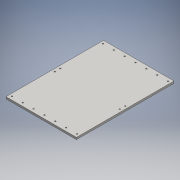
# Autodesk Inventor part: KrackenPlate1
Saved by Autodesk Inventor 2016 (Build 200138000, 138)
## iProperties
Created: 2015-09-06
Part Number: KrackenPlate1
Material: Generic
Document SubType Name: Modeling
Designer: Tim
Density: 1 g/cm^3
Appearance: Default
Author: Tim
Autodesk Inventor part; units mm, degrees
ref_plane "YZ Plane" through (0, 0, 0) normal (1, 0, 0) x (0, 1, 0)
ref_plane "XZ Plane" through (0, 0, 0) normal (0, 1, 0) x (-1, 0, 0)
ref_plane "XY Plane" through (0, 0, 0) normal (0, 0, 1) x (1, 0, 0)
sketch "Sketch1" plane through (0, 0, 0) normal (0, 0, 1) x (1, 0, 0)
  line L0 (104, -144) -> (-104, -144)
  line L1 (-104, -144) -> (-104, 144)
  line L2 (-104, 144) -> (104, 144)
  line L3 (104, 144) -> (104, -144)
  line L4 (104, -144) -> (-104, 144) construction
  line L5 (-104, -144) -> (104, 144) construction
  circle A0 centre (96, 134.4) radius 1.85
  circle A1 centre (64, 134.4) radius 1.85
  circle A2 centre (32, 134.4) radius 1.85
  circle A3 centre (0, 134.4) radius 1.85
  circle A4 centre (-32, 134.4) radius 1.85
  circle A5 centre (-64, 134.4) radius 1.85
  circle A6 centre (-96, 134.4) radius 1.85
  circle A7 centre (64, -134.4) radius 1.85
  circle A8 centre (32, -134.4) radius 1.85
  circle A9 centre (96, -134.4) radius 1.85
  circle A10 centre (0, -134.4) radius 1.85
  circle A11 centre (-32, -134.4) radius 1.85
  circle A12 centre (-96, -134.4) radius 1.85
  line L6 (104, 144) -> (-104, -144) construction
  line L7 (-104, 144) -> (104, -144) construction
  circle A13 centre (-64, -134.4) radius 1.85
  circle A14 centre (-96, 8) radius 1.85 projected
  circle A15 centre (-96, -8) radius 1.85 projected
  circle A16 centre (96, 8) radius 1.85 projected
  circle A17 centre (96, -8) radius 1.85 projected
  dimension "d0" = 208
  dimension "d1" = 288
  constraints: 16 end point, 2 parallel, 1 horizontal, 1 perpendicular
  measures "d0" distance of L2.start L2.end
  measures "d1" distance of L2.end L3.end
extrude "Extrusion5" add sketch "Sketch1" along normal blind 6
body "Solid5"
